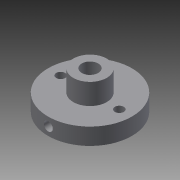
# Autodesk Inventor part: carousel_hub
Saved by Autodesk Inventor 2013 (Build 170138000, 138)
## iProperties
Created: 2013-07-26
Part Number: carousel_hub
Material: Generic
Document SubType Name: Modeling
Designer: dkboone
Density: 1 g/cm^3
Author: dkboone
Autodesk Inventor part; units mm, degrees
note: some values were not read from the file. Chosen so that the rebuilt part matches the saved one: direction of "Hole2".
ref_plane "YZ Plane" through (0, 0, 0) normal (1, 0, 0) x (0, 1, 0)
ref_plane "XZ Plane" through (0, 0, 0) normal (0, 1, 0) x (-1, 0, 0)
sketch "Sketch1" plane through (0, 0, 0) normal (0, 0, 1) x (1, 0, 0)
  line L0 (2.5, 11.43) -> (5.08, 11.43)
  line L1 (5.08, 11.43) -> (5.08, 5.08)
  line L2 (5.08, 5.08) -> (12.7, 5.08)
  line L3 (12.7, 5.08) -> (12.7, 0)
  line L4 (12.7, 0) -> (2.5, 0)
  line L5 (2.5, 0) -> (2.5, 11.43)
  line L6 (0, -2.286) -> (0, 13.716) projected
  point P0 (0, 0)
  dimension "d0" = 2.5
  dimension "d1" = 12.7
  dimension "d2" = 5.08
  dimension "d3" = 5.08
  dimension "d4" = 6.35
  constraints: 12 end point, 4 parallel, 1 horizontal, 1 perpendicular, 1 point on line
  measures "d0" distance from line of L5 point (0, 0)
  measures "d1" distance from line of point (0, 0) L3
  measures "d2" distance from line of point (0, 0) L1
  measures "d3" distance of L2.end L3.end
  measures "d4" distance of L0.end L1.end
revolve "Revolution1" add sketch "Sketch1" angle 360 about axis through (0, -10, 0) along (0, 1, 0)
sketch "Sketch2" plane through (0, 5.08, 0) normal (0, 1, 0) x (1, 0, 0)
  circle A0 centre (0, 0) radius 12.7 projected
  line L0 (-8.89, 0) -> (8.89, 0) construction
  dimension "d6" = 17.78
  constraints: 2 end point, 1 coincident, 1 horizontal, 1 midpoint
  measures "d6" distance of L0.start L0.end
hole "Hole1" at (-8.89, 5.08, 0) at (8.89, 5.08, 0) direction (0, -1, 0) diameter 2.7051 end through all
ref_plane "Work Plane1" through (0, 2.54, 12.7) normal (0, 0, 1) x (1, 0, 0)
sketch "Sketch3" plane through (0, 2.54, 12.7) normal (0, 0, 1) x (1, 0, 0)
  point P0 (0, -2.54)
  point P1 (0, 0)
  dimension "d17" = 2.54
  dimension "d18" = 0
  measures "d17" distance of point (0, 0) point (0, -2.54)
  measures "d18" horizontal distance of point (0, -2.54) point (0, 0)
hole "Hole2" at (0, 2.54, 12.7) direction (0, 0, -1) diameter 2.7051 end up to surface
body "Solid1"
